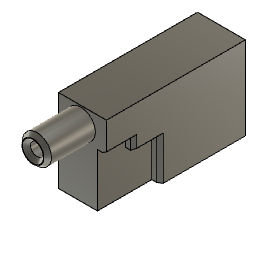
Nerf_gun (Autodesk Fusion 360 design; units mm, degrees)
Autodesk Fusion 360 part; units mm, degrees
sketch "Sketch1" plane through (0, 0, 0) normal (0, 1, 0) x (1, 0, 0)
  circle A0 centre (0, -75) radius 18.05
  circle A1 centre (0, -75) radius 8.05
  dimension "d1" = 36.1
  dimension "d6" = 16.1
  constraint concentric A0 A1
  measures "d1" diameter of A0
  measures "d6" diameter of A1
extrude "Extrude1" add sketch "Sketch1" along normal blind 230
chamfer "Chamfer1" distance 5 angle 40 1 edges at (-16.8285, 0, 81.5272) measured on face at (18.0276, 153.3333, 75.8997)
chamfer "Chamfer2" distance 5 angle 45 1 edges at (-7.5052, 0, 72.089)
ref_plane "WorkPlane1" through (0, 60, 0) normal (0, 1, 0) x (0, 0, 1)
sketch "Sketch2" plane through (0, 60, 0) normal (0, 1, 0) x (1, 0, 0)
  line L0 (31.9053, 9.0665) -> (-28.0947, 9.0665)
  line L1 (-28.0947, 9.0665) -> (-28.0947, -94.9335)
  line L2 (-28.0947, -94.9335) -> (31.9053, -94.9335)
  line L3 (31.9053, -94.9335) -> (31.9053, 9.0665)
  line L4 (31.9053, 9.0665) -> (-28.0947, -94.9335) construction
  line L5 (-28.0947, 9.0665) -> (31.9053, -94.9335) construction
  line L6 (-0.1401, -74.9335) -> (-63.0075, -74.9335) construction
  point P0 (1.9053, -42.9335)
  dimension "d9" = 60
  dimension "d10" = 104
  dimension "d11" = 20
  constraint horizontal L0
  constraint perpendicular L0 L1
  constraint parallel L0 L2
  constraint parallel L1 L3
  constraint coincident L4 P0
  constraint coincident L5 P0
  constraint perpendicular L1 L6
  measures "d9" distance of L1.end L2.end
  measures "d10" distance of L0.end L1.end
  measures "d11" distance of L2 L6
extrude "Extrude2" add sketch "Sketch2" along normal blind 174
sketch "Sketch3" plane through (31.9053, 0, 0) normal (1, 0, 0) x (0, 1, 0)
  line L0 (60, 94.9335) -> (60, -9.0665)
  line L1 (60, -9.0665) -> (234, -9.0665)
  line L2 (234, -9.0665) -> (234, 94.9335)
  line L3 (234, 94.9335) -> (60, 94.9335)
  line L4 (60, 57.4468) -> (234, 57.4468) construction
  line L5 (60, 75) -> (234, 75) construction
  line L6 (60, 57.4468) -> (95, 57.4468)
  line L7 (95, 57.4468) -> (95, 42.4468)
  line L8 (95, 42.4468) -> (128, 42.4468)
  line L9 (128, 42.4468) -> (128, -9.0665)
  line L10 (60, -9.0665) -> (60, 42.9335)
  dimension "d14" = 35
  dimension "d15" = 15
  dimension "d16" = 33
  constraint coincident L0 L4.start
  constraint coincident L2 L4.end
  constraint perpendicular L2 L4
  constraint coincident L0 L5.start
  constraint coincident L2 L5.end
  constraint perpendicular L2 L5
  constraint perpendicular L0 L6
  constraint perpendicular L4 L7
  constraint perpendicular L7 L8
  constraint coincident L1 L9.end
  constraint perpendicular L1 L9
  constraint coincident L0.end L1.start
  constraint midpoint L0 L10.end
  measures "d14" distance of L4.start L6.end
  measures "d15" distance of L6.end L7.end
  measures "d16" distance of L7.end L8.end
extrude "Extrude3" cut sketch "Sketch3" against normal blind 11.2 contours L0 L1 L6 L7 L8 L9 L10
chamfer "Chamfer3" distance 3 distance2 5 4 edges at (31.9053, 77.5, 57.4468) (31.9053, 95, 49.9468) (31.9053, 111.5, 42.4468) (31.9053, 128, 16.6901) measured on face at (31.9053, 198.6667, 42.7713) measured on face at (31.9053, 198.6667, 42.7713) measured on face at (31.9053, 198.6667, 42.7713) measured on face at (31.9053, 198.6667, 42.7713)
